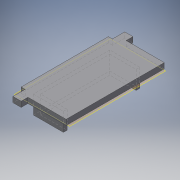
# Autodesk Inventor part: camera_holder
Saved by Autodesk Inventor 2018 (Build 220112000, 112)
## iProperties
Created: 2018-01-12
Part Number: camera_holder
Material: Generic
Document SubType Name: Modeling
Designer: erwin
Density: 1 g/cm^3
Appearance: Default
Author: erwin
Autodesk Inventor part; units mm, degrees
ref_plane "YZ Plane" through (0, 0, 0) normal (1, 0, 0) x (0, 1, 0)
ref_plane "XZ Plane" through (0, 0, 0) normal (0, 1, 0) x (-1, 0, 0)
ref_plane "XY Plane" through (0, 0, 0) normal (0, 0, 1) x (1, 0, 0)
ref_plane "Work Plane1" through (0, 0, 0) normal (0, 0, 1) x (1, 0, 0)
sketch "Sketch1" plane through (0, 0, 0) normal (0, 0, 1) x (1, 0, 0)
  line L0 (0, 0) -> (23.25, 0) projected
  line L1 (0, -48) -> (0, 0) projected
  line L2 (23.25, -48) -> (0, -48) projected
  line L3 (23.25, -48) -> (23.25, -31.5) projected
  line L4 (23.25, -31.5) -> (26.25, -31.5) projected
  line L5 (27.75, -30) -> (26.25, -31.5) projected
  line L6 (27.75, -30) -> (27.75, -18) projected
  line L7 (27.75, -18) -> (26.25, -16.5) projected
  line L8 (23.25, -16.5) -> (26.25, -16.5) projected
  line L9 (23.25, 0) -> (23.25, -16.5) projected
  line L10 (20.25, -16.5) -> (20.25, -3) projected
  line L11 (17.25, -16.5) -> (20.25, -16.5) projected
  line L12 (17.25, -16.5) -> (17.25, -19.5) projected
  line L13 (26.25, -19.5) -> (26.25, -28.5) projected
  line L14 (17.25, -28.5) -> (17.25, -31.5) projected
  line L15 (17.25, -31.5) -> (20.25, -31.5) projected
  line L16 (20.25, -31.5) -> (20.25, -45) projected
  line L17 (3.75, -45) -> (20.25, -45) projected
  line L18 (3.75, -3) -> (3.75, -45) projected
  line L19 (20.25, -3) -> (3.75, -3) projected
  line L20 (17.25, -19.5) -> (17.25, -28.5)
  line L21 (18.25, -33.5) -> (15.25, -33.5)
  line L22 (15.25, -33.5) -> (15.25, -28.5)
  line L23 (15.25, -28.5) -> (15.25, -19.5)
  line L24 (15.25, -19.5) -> (15.25, -14.5)
  line L25 (15.25, -14.5) -> (18.25, -14.5)
  line L26 (20.25, -5) -> (5.75, -5)
  line L27 (5.75, -5) -> (5.75, -43)
  line L28 (5.75, -43) -> (20.25, -43)
  constraints: 18 end point, 2 point on line, 1 vertical, 4 other
extrude "Extrusion1" add sketch "Sketch1" against normal blind 10 contours L26 L27 L28 L16 L17 L18 L19 L10
sketch "Sketch2" plane through (0, 0, 0) normal (0, 0, 1) x (1, 0, 0)
  line L0 (2.25, 0) -> (2.25, 6.75) projected
  line L1 (2.25, 0) -> (3.3, 0) projected
  line L2 (3.3, 0) -> (3.3, 5.7) projected
  line L3 (5.7, 5.7) -> (3.3, 5.7) projected
  line L4 (5.7, 1.95) -> (5.7, 5.7) projected
  line L5 (26.7, 1.95) -> (5.7, 1.95) projected
  line L6 (26.7, 1.95) -> (26.7, -16.95) projected
  line L7 (26.7, -16.95) -> (27.75, -18) projected
  line L8 (27.75, -18) -> (27.75, 3) projected
  line L9 (6.75, 3) -> (27.75, 3) projected
  line L10 (6.75, 3) -> (6.75, 6.75) projected
  line L11 (2.25, 6.75) -> (6.75, 6.75) projected
  line L12 (2.25, -54.75) -> (2.25, -48) projected
  line L13 (2.25, -54.75) -> (6.75, -54.75) projected
  line L14 (6.75, -54.75) -> (6.75, -51) projected
  line L15 (6.75, -51) -> (27.75, -51) projected
  line L16 (27.75, -51) -> (27.75, -30) projected
  line L17 (26.7, -31.05) -> (27.75, -30) projected
  line L18 (26.7, -31.05) -> (26.7, -49.95) projected
  line L19 (26.7, -49.95) -> (5.7, -49.95) projected
  line L20 (5.7, -49.95) -> (5.7, -53.7) projected
  line L21 (3.3, -53.7) -> (5.7, -53.7) projected
  line L22 (3.3, -53.7) -> (3.3, -48) projected
  line L23 (2.25, -48) -> (3.3, -48) projected
  line L24 (0, 0) -> (23.25, 0) projected
  line L25 (0, -48) -> (0, 0) projected
  line L26 (23.25, -48) -> (0, -48) projected
  line L27 (23.25, -48) -> (23.25, -31.5) projected
  line L28 (23.25, -31.5) -> (26.25, -31.5) projected
  line L29 (27.75, -30) -> (26.25, -31.5) projected
  line L30 (27.75, -30) -> (27.75, -18) projected
  line L31 (27.75, -18) -> (26.25, -16.5) projected
  line L32 (23.25, -16.5) -> (26.25, -16.5) projected
  line L33 (23.25, 0) -> (23.25, -16.5) projected
  line L34 (20.25, -16.5) -> (20.25, -3) projected
  line L35 (17.25, -16.5) -> (20.25, -16.5) projected
  line L36 (17.25, -16.5) -> (17.25, -19.5) projected
  line L37 (17.25, -19.5) -> (26.25, -19.5) projected
  line L38 (26.25, -19.5) -> (26.25, -28.5) projected
  line L39 (17.25, -28.5) -> (26.25, -28.5) projected
  line L40 (17.25, -28.5) -> (17.25, -31.5) projected
  line L41 (17.25, -31.5) -> (20.25, -31.5) projected
  line L42 (20.25, -31.5) -> (20.25, -45) projected
  line L43 (3.75, -45) -> (20.25, -45) projected
  line L44 (3.75, -3) -> (3.75, -45) projected
  line L45 (20.25, -3) -> (3.75, -3) projected
extrude "Extrusion2" add sketch "Sketch2" along normal blind 3 contours L0 L11 L10 L9 L8 L7 L6 L5 L4 L3 L2 L1 | L1 L24 L33 L32 L31 L7 L30 L17 L29 L28 L27 L26 L23 L25 | L2 L3 L4 L5 L6 L31 L32 L33 L24 | L23 L22 L21 L20 L19 L18 L17 L16 L15 L14 L13 L12 | L26 L27 L28 L29 L18 L19 L20 L21 L22 | L35 L36 L37 L38 L39 L40 L41 L42 L43 L44 L45 L34
sketch "Sketch3" plane through (0, 0, 0) normal (0, 0, -1) x (-1, 0, 0)
  line L0 (-5.75, -34) -> (-15.75, -34)
  line L1 (-15.75, -34) -> (-15.75, -14)
  line L2 (-15.75, -14) -> (-5.75, -14)
  line L3 (-5.75, -14) -> (-5.75, -34)
  line L4 (-3.75, -45) -> (-3.75, -3) construction
  line L5 (-3.75, -24) -> (-33.6662, -24) construction
  line L6 (-5.75, -5) -> (-5.75, -43) construction
  point P0 (0, 0)
  dimension "d5" = 10
  dimension "d6" = 20
  constraints: 10 end point, 2 horizontal, 2 parallel, 1 collinear, 1 midpoint, 1 perpendicular, 1 other
  measures "d5" distance of L1.end L2.end
  measures "d6" distance of L0.end L1.end
extrude "Extrusion3" cut sketch "Sketch3" against normal through all
sketch "Sketch4" plane through (0, 0, 0) normal (0, 0, -1) x (-1, 0, 0)
  line L0 (-20.25, -5) -> (-5.75, -5) projected
  line L1 (-5.75, -43) -> (-20.25, -43) projected
  line L2 (-5.75, -5) -> (-5.75, -43) projected
  point P0 (0, 0)
  point P1 (-9.75, -9)
  point P2 (-9.75, -39)
  dimension "d9" = 4
  dimension "d10" = 4
  dimension "d11" = 4
  dimension "d12" = 4
  measures "d9" distance from line of L0 point (-9.75, -9)
  measures "d10" distance from line of L1 point (-9.75, -39)
  measures "d11" distance from line of L2 point (-9.75, -39)
  measures "d12" distance from line of L2 point (-9.75, -9)
hole "Hole1" at (9.75, -9, 0) at (9.75, -39, 0) direction (0, 0, 1) diameter 3 end through all
fillet "Fillet1" radius 2 6 edges at (20.25, -4, -10) (20.25, -44, -10) (3.75, -3, -5) (3.75, -45, -5) (5.75, -43, -5) (5.75, -5, -5)
thicken "Thicken1" operation add thickness 0.1 both sides no extend neighbours yes toward (0, 1, 0) faces at (14.75, -45, -3.3333) (4.75, -44.732, -3.3333) (3.75, -17.6667, -3.3333) (4.2839, -3.6397, -3.3333) (14.75, -3, -3.3333)
equation "\"d12\" = d11"
body "Solid1"
